Autodesk Inventor part; units mm, degrees
(part 2 of 3)
sketch "Sketch8" plane through (0, 0, 6.35) normal (0, 0, 1) x (1, 0, 0)
  line L0 (-60.6619, -189.7645) -> (-88.5384, -146.9458) projected
  arc A0 (-88.5384, -146.9458) -> (-92.3643, -145.7246) centre (-91.1992, -148.6781) ccw projected
  arc A1 (-96.1321, -146.5792) -> (-92.3643, -145.7246) centre (-97.0248, -133.9106) ccw projected
  arc A2 (-96.1321, -146.5792) -> (-99.0202, -149.1135) centre (-95.909, -149.7463) ccw projected
  line L1 (-99.0202, -149.1135) -> (-103.0485, -168.9169) projected
  arc A3 (-103.0485, -168.9169) -> (-101.38, -172.378) centre (-99.9372, -169.5497) ccw projected
  arc A4 (-94.5438, -182.1572) -> (-101.38, -172.378) centre (-107.1508, -183.6911) ccw projected
  arc A5 (-94.5438, -182.1572) -> (-92.4345, -184.7727) centre (-91.3921, -181.7737) ccw projected
  line L2 (-92.4345, -184.7727) -> (-64.3902, -194.5205) projected
  arc A6 (-64.3902, -194.5205) -> (-61.1133, -193.7771) centre (-63.3478, -191.5215) ccw projected
  arc A7 (-61.0933, -193.7573) -> (-61.1133, -193.7771) centre (-52.1756, -202.7997) ccw projected
  arc A8 (-61.0933, -193.7573) -> (-60.6619, -189.7645) centre (-63.3227, -191.4968) ccw projected
  line L3 (-39.1869, -128.4485) -> (-78.3293, -96.1428) projected
  arc A9 (-86.006, -96.7986) -> (-81.66, -95.6992) centre (-86.8987, -84.1301) ccw projected
  arc A10 (-86.006, -96.7986) -> (-88.8942, -99.3329) centre (-85.7829, -99.9658) ccw projected
  line L4 (-88.8942, -99.3329) -> (-92.9225, -119.1363) projected
  arc A11 (-92.9225, -119.1363) -> (-91.2539, -122.5975) centre (-89.8112, -119.7692) ccw projected
  arc A12 (-85.2508, -129.1499) -> (-91.2539, -122.5975) centre (-97.0248, -133.9106) ccw projected
  arc A13 (-85.2508, -129.1499) -> (-82.5337, -131.1266) centre (-82.3074, -127.9597) ccw projected
  line L5 (-82.5337, -131.1266) -> (-51.925, -133.3143) projected
  arc A14 (-49.8906, -133.4597) -> (-51.925, -133.3143) centre (-51.8103, -146.0138) ccw projected
  line L6 (-49.8906, -133.4597) -> (-41.4343, -134.0641) projected
  arc A15 (-41.4343, -134.0641) -> (-39.1869, -128.4485) centre (-41.2079, -130.8972) ccw projected
  line L7 (-34.396, -142.2066) -> (-35.726, -142.1115) projected
  arc A16 (-35.726, -142.1115) -> (-39.1239, -145.4255) centre (-35.9523, -145.2784) ccw projected
  arc A17 (-46.8246, -157.6942) -> (-39.1239, -145.4255) centre (-51.8103, -146.0138) ccw projected
  line L8 (-46.8246, -157.6942) -> (-63.3432, -164.745) projected
  arc A18 (-63.388, -164.764) -> (-63.3432, -164.745) centre (-68.3289, -153.0646) ccw projected
  arc A19 (-63.388, -164.764) -> (-64.8136, -169.4212) centre (-62.1528, -167.6889) ccw projected
  line L9 (-64.8136, -169.4212) -> (-52.1403, -188.8876) projected
  arc A20 (-52.1403, -188.8876) -> (-50.0187, -190.2842) centre (-49.4795, -187.1553) ccw projected
  arc A21 (-49.6531, -190.3527) -> (-50.0187, -190.2842) centre (-52.1756, -202.7997) ccw projected
  arc A22 (-49.6531, -190.3527) -> (-46.1932, -188.6816) centre (-49.0225, -187.241) ccw projected
  line L10 (-46.1932, -188.6816) -> (-27.8032, -152.5651) projected
  arc A23 (-27.8032, -152.5651) -> (-28.487, -148.784) centre (-30.6326, -151.1244) ccw projected
  arc A24 (-31.6788, -144.1833) -> (-28.487, -148.784) centre (-19.9049, -139.4226) ccw projected
  arc A25 (-31.6788, -144.1833) -> (-34.396, -142.2066) centre (-34.6223, -145.3735) ccw projected
  circle A26 centre (-19.9049, -139.4226) radius 5.588 projected
  circle A27 centre (12.3657, -76.0454) radius 5.588 projected
  circle A28 centre (-52.1756, -202.7997) radius 5.588 projected
  circle A29 centre (-10.4424, -25.9152) radius 6.731 projected
  circle A30 centre (-6.7845, 27.1038) radius 6.731 projected
  line L11 (-56.4256, -250.7609) -> (56.5867, -28.8131) projected
  arc A31 (-133.6537, -223.8049) -> (-56.4256, -250.7609) centre (-93.207, -232.0324) ccw projected
  line L12 (-94.3869, -30.7665) -> (-133.6537, -223.8049) projected
  arc A32 (-79.8174, 0.8875) -> (-94.3869, -30.7665) centre (-19.7161, -45.9556) ccw projected
  line L13 (-50.0844, 39.0359) -> (-79.8174, 0.8875) projected
  arc A33 (56.5867, -28.8131) -> (-50.0844, 39.0359) centre (0, 0) ccw projected
  circle A34 centre (0, 0) radius 13.4937 projected
  line L14 (-92.6277, -239.1082) -> (-87.8938, -227.3235) projected
  arc A35 (-87.8938, -227.3235) -> (-93.7862, -224.9565) centre (-90.84, -226.14) ccw projected
  line L15 (-93.7862, -224.9565) -> (-98.5201, -236.7413) projected
  arc A36 (-98.5201, -236.7413) -> (-92.6277, -239.1082) centre (-95.5739, -237.9247) ccw projected
  circle A37 centre (23.6807, 14.828) radius 6.731 projected
  circle A38 centre (-27.8737, 1.9231) radius 6.731 projected
  circle A39 centre (21.42, -17.9396) radius 6.731 projected
  arc A40 (-106.2582, -196.3597) -> (-98.2131, -192.7137) centre (-107.1508, -183.6911) ccw projected
  arc A41 (-106.2582, -196.3597) -> (-109.1463, -198.894) centre (-106.035, -199.5269) ccw projected
  line L16 (-109.1463, -198.894) -> (-109.9229, -202.7119) projected
  arc A42 (-109.9229, -202.7119) -> (-105.4512, -206.2136) centre (-106.8116, -203.3448) ccw projected
  arc A43 (-67.5559, -219.4407) -> (-76.9832, -208.5096) centre (-93.207, -232.0324) ccw projected
  arc A44 (-67.5559, -219.4407) -> (-61.8764, -219.4822) centre (-64.7057, -218.0416) ccw projected
  line L17 (-61.8764, -219.4822) -> (-60.0739, -215.9422) projected
  arc A45 (-60.0739, -215.9422) -> (-60.7577, -212.1612) centre (-62.9032, -214.5015) ccw projected
  arc A46 (-64.7826, -204.3336) -> (-60.7577, -212.1612) centre (-52.1756, -202.7997) ccw projected
  arc A47 (-64.7826, -204.3336) -> (-66.8919, -201.7181) centre (-67.9343, -204.7171) ccw projected
  line L18 (-66.8919, -201.7181) -> (-72.8348, -199.6524) projected
  arc A48 (-94.9362, -191.9703) -> (-98.2131, -192.7137) centre (-95.9786, -194.9693) ccw projected
  line L19 (-62.2455, -36.9386) -> (-28.8338, -52.5675) projected
  arc A49 (1.0672, -66.5541) -> (4.4031, -66.1517) centre (2.4124, -63.6782) ccw projected
  arc A50 (14.8881, -63.5984) -> (4.4031, -66.1517) centre (12.3657, -76.0454) ccw projected
  arc A51 (14.8881, -63.5984) -> (18.3481, -61.9274) centre (15.5187, -60.4867) ccw projected
  line L20 (18.3481, -61.9274) -> (26.6737, -45.5765) projected
  arc A52 (26.6737, -45.5765) -> (22.3352, -41.3425) centre (23.8443, -44.1359) ccw projected
  arc A53 (-11.2735, -45.6176) -> (22.3352, -41.3425) centre (0, 0) ccw projected
  arc A54 (-46.9122, 2.7029) -> (-52.5862, 4.8373) centre (-50.0819, 2.8855) ccw projected
  line L21 (-52.5862, 4.8373) -> (-64.7921, -10.8233) projected
  arc A55 (-64.7921, -10.8233) -> (-70.5555, -19.8506) centre (-19.7161, -45.9556) ccw projected
  arc A56 (-70.5555, -19.8506) -> (-69.5394, -23.9106) centre (-67.7311, -21.3009) ccw projected
  arc A57 (-64.0747, -34.1201) -> (-69.5394, -23.9106) centre (-76.7726, -34.3495) ccw projected
  arc A58 (-64.0747, -34.1201) -> (-62.2455, -36.9386) centre (-60.9002, -34.0627) ccw projected
  arc A59 (-75.88, -47.0181) -> (-68.81, -44.2433) centre (-76.7726, -34.3495) ccw projected
  arc A60 (-75.88, -47.0181) -> (-78.7681, -49.5524) centre (-75.6568, -50.1853) ccw projected
  line L22 (-78.7681, -49.5524) -> (-82.7964, -69.3558) projected
  arc A61 (-82.7964, -69.3558) -> (-81.1278, -72.8169) centre (-79.6851, -69.9886) ccw projected
  arc A62 (-75.9854, -77.6347) -> (-81.1278, -72.8169) centre (-86.8987, -84.1301) ccw projected
  arc A63 (-75.9854, -77.6347) -> (-72.9993, -79.1754) centre (-73.2571, -76.0109) ccw projected
  line L23 (-72.9993, -79.1754) -> (-14.1778, -74.3847) projected
  arc A64 (-14.1778, -74.3847) -> (-13.0902, -68.3442) centre (-14.4355, -71.2201) ccw projected
  line L24 (-13.0902, -68.3442) -> (-65.4741, -43.8408) projected
  arc A65 (-65.4741, -43.8408) -> (-68.81, -44.2433) centre (-66.8194, -46.7167) ccw projected
  arc A66 (-17.3825, -126.9756) -> (-25.1437, -127.8534) centre (-19.9049, -139.4226) ccw projected
  arc A67 (-17.3825, -126.9756) -> (-13.9226, -125.3045) centre (-16.7519, -123.8638) ccw projected
  line L25 (-13.9226, -125.3045) -> (4.4674, -89.1879) projected
  arc A68 (4.4674, -89.1879) -> (3.7836, -85.4069) centre (1.6381, -87.7473) ccw projected
  arc A69 (1.4524, -82.5408) -> (3.7836, -85.4069) centre (12.3657, -76.0454) ccw projected
  arc A70 (1.4524, -82.5408) -> (-1.5337, -81.0001) centre (-1.2759, -84.1646) ccw projected
  line L26 (-1.5337, -81.0001) -> (-69.4401, -86.5307) projected
  arc A71 (-69.4401, -86.5307) -> (-71.2033, -92.144) centre (-69.1823, -89.6953) ccw projected
  line L27 (-71.2033, -92.144) -> (-28.4744, -127.4098) projected
  arc A72 (-28.4744, -127.4098) -> (-25.1437, -127.8534) centre (-26.4534, -124.9611) ccw projected
  circle A73 centre (-68.3289, -153.0646) radius 6.731 projected
  circle A74 centre (-51.8103, -146.0138) radius 6.731 projected
  line L28 (-76.8234, -201.468) -> (-78.1267, -204.7125) projected
  line L29 (-16.1602, -58.4958) -> (1.0672, -66.5541) projected
  line L30 (-14.9814, -47.5164) -> (-17.7611, -54.4364) projected
  line L31 (-85.1976, -201.8722) -> (-84.1415, -199.2432) projected
  line L32 (-86.0453, -195.0607) -> (-94.9362, -191.9703) projected
  arc A75 (-88.6501, -203.823) -> (-105.4512, -206.2136) centre (-93.207, -232.0324) ccw projected
  line L33 (-24.5423, -50.875) -> (-22.0522, -44.6761) projected
  arc A76 (-46.9122, 2.7029) -> (-23.4162, -40.7399) centre (0, 0) ccw projected
  arc A77 (-72.8348, -199.6524) -> (-76.8234, -201.468) centre (-73.8772, -202.6514) ccw projected
  arc A78 (-78.1267, -204.7125) -> (-76.9832, -208.5096) centre (-75.1805, -205.896) ccw projected
  arc A79 (-11.2735, -45.6176) -> (-14.9814, -47.5164) centre (-12.0352, -48.6999) ccw projected
  arc A80 (-17.7611, -54.4364) -> (-16.1602, -58.4958) centre (-14.8149, -55.6198) ccw projected
  arc A81 (-78.3293, -96.1428) -> (-81.66, -95.6992) centre (-80.3503, -98.5915) ccw projected
  arc A82 (-84.1415, -199.2432) -> (-86.0453, -195.0607) centre (-87.0877, -198.0597) ccw projected
  arc A83 (-88.6501, -203.823) -> (-85.1976, -201.8722) centre (-88.1438, -200.6887) ccw projected
  arc A84 (-22.0522, -44.6761) -> (-23.4162, -40.7399) centre (-24.9984, -43.4926) ccw projected
  arc A85 (-28.8338, -52.5675) -> (-24.5423, -50.875) centre (-27.4885, -49.6916) ccw projected
  point P0 (0, 0)
  point P1 (-93.2076, -232.0321)
  point P2 (0, 0)
extrude "Extrusion8" cut sketch "Sketch8" against normal blind 6.35 contours A8 A7 A6 L2 A5 A4 A3 L1 A2 A1 A0 L0 | A40 A48 L32 A82 L31 A83 A75 A42 L16 A41 | A43 A78 L28 A77 L18 A47 A46 A45 L17 A44 | A58 A57 A56 A55 L21 A54 A76 A84 L33 A85 L19 | L29 A80 L30 A79 A53 A52 L20 A51 A50 A49 | A59 A65 L24 A64 L23 A63 A62 A61 L22 A60 | A66 A72 L27 A71 L26 A70 A69 A68 L25 A67
sketch "Sketch9" plane through (0, 0, 6.35) normal (0, 0, 1) x (1, 0, 0)
  arc A0 (-88.6501, -203.823) -> (-105.4512, -206.2136) centre (-93.207, -232.0324) ccw projected
  arc A1 (-109.9229, -202.7119) -> (-105.4512, -206.2136) centre (-106.8116, -203.3448) ccw projected
  line L0 (-109.9229, -202.7119) -> (-109.1463, -198.894) projected
  arc A2 (-106.2582, -196.3597) -> (-109.1463, -198.894) centre (-106.035, -199.5269) ccw projected
  arc A3 (-106.2582, -196.3597) -> (-98.2131, -192.7137) centre (-107.1508, -183.6911) ccw projected
  arc A4 (-94.9362, -191.9703) -> (-98.2131, -192.7137) centre (-95.9786, -194.9693) ccw projected
  line L1 (-94.9362, -191.9703) -> (-86.0453, -195.0607) projected
  arc A5 (-84.1415, -199.2432) -> (-86.0453, -195.0607) centre (-87.0877, -198.0597) ccw projected
  line L2 (-84.1415, -199.2432) -> (-85.1976, -201.8722) projected
  arc A6 (-88.6501, -203.823) -> (-85.1976, -201.8722) centre (-88.1438, -200.6887) ccw projected
  arc A7 (-28.8338, -52.5675) -> (-24.5423, -50.875) centre (-27.4885, -49.6916) ccw projected
  line L3 (-28.8338, -52.5675) -> (-62.2455, -36.9386) projected
  arc A8 (-64.0747, -34.1201) -> (-62.2455, -36.9386) centre (-60.9002, -34.0627) ccw projected
  arc A9 (-64.0747, -34.1201) -> (-69.5394, -23.9106) centre (-76.7726, -34.3495) ccw projected
  arc A10 (-70.5555, -19.8506) -> (-69.5394, -23.9106) centre (-67.7311, -21.3009) ccw projected
  arc A11 (-64.7921, -10.8233) -> (-70.5555, -19.8506) centre (-19.7161, -45.9556) ccw projected
  line L4 (-64.7921, -10.8233) -> (-52.5862, 4.8373) projected
  arc A12 (-46.9122, 2.7029) -> (-52.5862, 4.8373) centre (-50.0819, 2.8855) ccw projected
  arc A13 (-46.9122, 2.7029) -> (-23.4162, -40.7399) centre (0, 0) ccw projected
  arc A14 (-22.0522, -44.6761) -> (-23.4162, -40.7399) centre (-24.9984, -43.4926) ccw projected
  line L5 (-22.0522, -44.6761) -> (-24.5423, -50.875) projected
  arc A15 (-88.5384, -146.9458) -> (-92.3643, -145.7246) centre (-91.1992, -148.6781) ccw projected
  line L6 (-88.5384, -146.9458) -> (-60.6619, -189.7645) projected
  arc A16 (-61.0933, -193.7573) -> (-60.6619, -189.7645) centre (-63.3227, -191.4968) ccw projected
  arc A17 (-61.0933, -193.7573) -> (-61.1133, -193.7771) centre (-52.1756, -202.7997) ccw projected
  arc A18 (-64.3902, -194.5205) -> (-61.1133, -193.7771) centre (-63.3478, -191.5215) ccw projected
  line L7 (-64.3902, -194.5205) -> (-92.4345, -184.7727) projected
  arc A19 (-94.5438, -182.1572) -> (-92.4345, -184.7727) centre (-91.3921, -181.7737) ccw projected
  arc A20 (-94.5438, -182.1572) -> (-101.38, -172.378) centre (-107.1508, -183.6911) ccw projected
  arc A21 (-103.0485, -168.9169) -> (-101.38, -172.378) centre (-99.9372, -169.5497) ccw projected
  line L8 (-103.0485, -168.9169) -> (-99.0202, -149.1135) projected
  arc A22 (-96.1321, -146.5792) -> (-99.0202, -149.1135) centre (-95.909, -149.7463) ccw projected
  arc A23 (-96.1321, -146.5792) -> (-92.3643, -145.7246) centre (-97.0248, -133.9106) ccw projected
  arc A24 (-17.7611, -54.4364) -> (-16.1602, -58.4958) centre (-14.8149, -55.6198) ccw projected
  line L9 (-17.7611, -54.4364) -> (-14.9814, -47.5164) projected
  arc A25 (-11.2735, -45.6176) -> (-14.9814, -47.5164) centre (-12.0352, -48.6999) ccw projected
  arc A26 (-11.2735, -45.6176) -> (22.3352, -41.3425) centre (0, 0) ccw projected
  arc A27 (26.6737, -45.5765) -> (22.3352, -41.3425) centre (23.8443, -44.1359) ccw projected
  line L10 (26.6737, -45.5765) -> (18.3481, -61.9274) projected
  arc A28 (14.8881, -63.5984) -> (18.3481, -61.9274) centre (15.5187, -60.4867) ccw projected
  arc A29 (14.8881, -63.5984) -> (4.4031, -66.1517) centre (12.3657, -76.0454) ccw projected
  arc A30 (1.0672, -66.5541) -> (4.4031, -66.1517) centre (2.4124, -63.6782) ccw projected
  line L11 (1.0672, -66.5541) -> (-16.1602, -58.4958) projected
  arc A31 (-75.9854, -77.6347) -> (-81.1278, -72.8169) centre (-86.8987, -84.1301) ccw projected
  arc A32 (-82.7964, -69.3558) -> (-81.1278, -72.8169) centre (-79.6851, -69.9886) ccw projected
  line L12 (-82.7964, -69.3558) -> (-78.7681, -49.5524) projected
  arc A33 (-75.88, -47.0181) -> (-78.7681, -49.5524) centre (-75.6568, -50.1853) ccw projected
  arc A34 (-75.88, -47.0181) -> (-68.81, -44.2433) centre (-76.7726, -34.3495) ccw projected
  arc A35 (-65.4741, -43.8408) -> (-68.81, -44.2433) centre (-66.8194, -46.7167) ccw projected
  line L13 (-65.4741, -43.8408) -> (-13.0902, -68.3442) projected
  arc A36 (-14.1778, -74.3847) -> (-13.0902, -68.3442) centre (-14.4355, -71.2201) ccw projected
  line L14 (-14.1778, -74.3847) -> (-72.9993, -79.1754) projected
  arc A37 (-75.9854, -77.6347) -> (-72.9993, -79.1754) centre (-73.2571, -76.0109) ccw projected
  arc A38 (1.4524, -82.5408) -> (3.7836, -85.4069) centre (12.3657, -76.0454) ccw projected
  arc A39 (4.4674, -89.1879) -> (3.7836, -85.4069) centre (1.6381, -87.7473) ccw projected
  line L15 (4.4674, -89.1879) -> (-13.9226, -125.3045) projected
  arc A40 (-17.3825, -126.9756) -> (-13.9226, -125.3045) centre (-16.7519, -123.8638) ccw projected
  arc A41 (-17.3825, -126.9756) -> (-25.1437, -127.8534) centre (-19.9049, -139.4226) ccw projected
  arc A42 (-28.4744, -127.4098) -> (-25.1437, -127.8534) centre (-26.4534, -124.9611) ccw projected
  line L16 (-28.4744, -127.4098) -> (-71.2033, -92.144) projected
  arc A43 (-69.4401, -86.5307) -> (-71.2033, -92.144) centre (-69.1823, -89.6953) ccw projected
  line L17 (-69.4401, -86.5307) -> (-1.5337, -81.0001) projected
  arc A44 (1.4524, -82.5408) -> (-1.5337, -81.0001) centre (-1.2759, -84.1646) ccw projected
  arc A45 (-64.7826, -204.3336) -> (-60.7577, -212.1612) centre (-52.1756, -202.7997) ccw projected
  arc A46 (-60.0739, -215.9422) -> (-60.7577, -212.1612) centre (-62.9032, -214.5015) ccw projected
  line L18 (-60.0739, -215.9422) -> (-61.8764, -219.4822) projected
  arc A47 (-67.5559, -219.4407) -> (-61.8764, -219.4822) centre (-64.7057, -218.0416) ccw projected
  arc A48 (-67.5559, -219.4407) -> (-76.9832, -208.5096) centre (-93.207, -232.0324) ccw projected
  arc A49 (-78.1267, -204.7125) -> (-76.9832, -208.5096) centre (-75.1805, -205.896) ccw projected
  line L19 (-78.1267, -204.7125) -> (-76.8234, -201.468) projected
  arc A50 (-72.8348, -199.6524) -> (-76.8234, -201.468) centre (-73.8772, -202.6514) ccw projected
  line L20 (-72.8348, -199.6524) -> (-66.8919, -201.7181) projected
  arc A51 (-64.7826, -204.3336) -> (-66.8919, -201.7181) centre (-67.9343, -204.7171) ccw projected
  circle A52 centre (-19.9049, -139.4226) radius 5.588 projected
  circle A53 centre (-107.1541, -183.6919) radius 5.588 projected
  circle A54 centre (-86.902, -84.1308) radius 5.588 projected
  circle A55 centre (-56.5442, -157.7985) radius 6.731 projected
  line L21 (-98.5201, -236.7413) -> (-93.7862, -224.9565) projected
  arc A56 (-87.8938, -227.3235) -> (-93.7862, -224.9565) centre (-90.84, -226.14) ccw projected
  line L22 (-87.8938, -227.3235) -> (-92.6277, -239.1082) projected
  arc A57 (-98.5201, -236.7413) -> (-92.6277, -239.1082) centre (-95.5739, -237.9247) ccw projected
  circle A58 centre (0, 0) radius 13.4937 projected
  arc A59 (56.5867, -28.8131) -> (-50.0844, 39.0359) centre (0, 0) ccw projected
  line L23 (-50.0844, 39.0359) -> (-79.8174, 0.8875) projected
  arc A60 (-79.8174, 0.8875) -> (-94.3869, -30.7665) centre (-19.7161, -45.9556) ccw projected
  line L24 (-94.3869, -30.7665) -> (-133.6537, -223.8049) projected
  arc A61 (-133.6537, -223.8049) -> (-56.4256, -250.7609) centre (-93.207, -232.0324) ccw projected
  line L25 (-56.4256, -250.7609) -> (56.5867, -28.8131) projected
  circle A62 centre (-63.595, -141.2799) radius 6.731 projected
  arc A63 (-11.6087, -28.8683) -> (-9.2396, -22.9769) centre (-10.4059, -25.9299) ccw projected
  arc A64 (-9.2396, -22.9769) -> (-11.6087, -28.8683) centre (-10.4424, -25.9152) ccw projected
  arc A65 (26.36, 16.5315) -> (20.9805, 13.1578) centre (23.6598, 14.8613) ccw projected
  arc A66 (20.9805, 13.1578) -> (26.36, 16.5315) centre (23.6807, 14.828) ccw projected
  arc A67 (23.8681, -19.9613) -> (18.9971, -15.8876) centre (21.4452, -17.9094) ccw projected
  arc A68 (18.9971, -15.8876) -> (23.8681, -19.9613) centre (21.42, -17.9396) ccw projected
  arc A69 (-7.5767, 30.1783) -> (-6.0305, 24.0196) centre (-6.8227, 27.0942) ccw projected
  arc A70 (-6.0305, 24.0196) -> (-7.5767, 30.1783) centre (-6.7845, 27.1038) ccw projected
  arc A71 (-31.0426, 2.1197) -> (-24.7075, 1.6871) centre (-27.8764, 1.8838) ccw projected
  arc A72 (-24.7075, 1.6871) -> (-31.0426, 2.1197) centre (-27.8737, 1.9231) ccw projected
  circle A73 centre (-76.7759, -34.3502) radius 5.588 projected
  circle A74 centre (-97.0281, -133.9113) radius 5.588 projected
  circle A75 centre (12.3657, -76.0454) radius 5.588 projected
  circle A76 centre (-52.1756, -202.7997) radius 5.588 projected
  circle A77 centre (-56.5442, -157.7985) radius 3.175 projected
  circle A78 centre (-56.5442, -157.7985) radius 12.7
  circle A79 centre (-63.595, -141.2799) radius 12.7
  line L26 (-68.2246, -162.7842) -> (-75.2755, -146.2655)
  line L27 (-51.9146, -136.2942) -> (-44.8637, -152.8128)
  circle A80 centre (-19.9049, -139.4226) radius 2.413 projected
  circle A81 centre (-97.0281, -133.9113) radius 2.413 projected
  line L28 (-19.9049, -139.4226) -> (-97.0281, -133.9113)
  circle A82 centre (-52.1756, -202.7997) radius 2.413 projected
  line L29 (-97.0281, -133.9113) -> (-52.1756, -202.7997)
  line L30 (-57.469, -187.6858) -> (-85.3454, -144.8671)
  arc A83 (-85.3454, -144.8671) -> (-93.7625, -142.1804) centre (-91.1992, -148.6781) ccw
  arc A84 (-96.3999, -142.7786) -> (-93.7625, -142.1804) centre (-97.0248, -133.9106) ccw
  arc A85 (-96.3999, -142.7786) -> (-102.7538, -148.354) centre (-95.909, -149.7463) ccw
  line L31 (-102.7538, -148.354) -> (-106.7821, -168.1574)
  arc A86 (-106.7821, -168.1574) -> (-103.1112, -175.772) centre (-99.9372, -169.5497) ccw
  arc A87 (-98.3259, -182.6174) -> (-103.1112, -175.772) centre (-107.1508, -183.6911) ccw
  arc A88 (-98.3259, -182.6174) -> (-93.6854, -188.3715) centre (-91.3921, -181.7737) ccw
  line L32 (-93.6854, -188.3715) -> (-65.641, -198.1193)
  arc A89 (-65.641, -198.1193) -> (-58.432, -196.4839) centre (-63.3478, -191.5215) ccw
  arc A90 (-58.418, -196.47) -> (-58.432, -196.4839) centre (-52.1756, -202.7997) ccw
  arc A91 (-58.418, -196.47) -> (-57.469, -187.6858) centre (-63.3227, -191.4968) ccw
  line L33 (-19.647, -135.6213) -> (-104.4046, -129.5645)
  line L34 (-104.4046, -129.5645) -> (-55.3622, -204.8881)
  line L35 (-20.1902, -143.2219) -> (-89.6515, -138.2582)
  line L36 (-89.6515, -138.2582) -> (-48.9765, -200.7304)
  arc A92 (39.6107, -20.1691) -> (-35.0591, 27.3251) centre (0, 0) ccw
  line L37 (-35.0591, 27.3251) -> (-64.7921, -10.8233)
  arc A93 (-64.7921, -10.8233) -> (-75.7192, -34.5638) centre (-19.7161, -45.9556) ccw
  line L38 (-75.7192, -34.5638) -> (-114.986, -227.6022)
  arc A94 (-114.986, -227.6022) -> (-73.4016, -242.1169) centre (-93.207, -232.0324) ccw
  line L39 (-73.4016, -242.1169) -> (39.6107, -20.1691)
  line L40 (-76.0538, -98.0209) -> (-33.3248, -133.2867)
  arc A95 (-33.3248, -133.2867) -> (-22.0004, -134.7949) centre (-26.4534, -124.9611) ccw
  arc A96 (-18.896, -134.4438) -> (-22.0004, -134.7949) centre (-19.9049, -139.4226) ccw
  arc A97 (-18.896, -134.4438) -> (-7.1321, -128.762) centre (-16.7519, -123.8638) ccw
  line L41 (-7.1321, -128.762) -> (11.2578, -92.6455)
  arc A98 (11.2578, -92.6455) -> (8.9329, -79.79) centre (1.6381, -87.7473) ccw
  arc A99 (8.0004, -78.6436) -> (8.9329, -79.79) centre (12.3657, -76.0454) ccw
  arc A100 (8.0004, -78.6436) -> (-2.1522, -73.4052) centre (-1.2759, -84.1646) ccw
  line L42 (-2.1522, -73.4052) -> (-70.0586, -78.9359)
  arc A101 (-70.0586, -78.9359) -> (-76.0538, -98.0209) centre (-69.1823, -89.6953) ccw
  spline S0 degree 4 poles (-63.6057, -178.2615) (-65.5406, -175.2881) (-67.0528, -169.1426) (-60.675, -170.3492) (-57.0315, -170.4891) knots 0 0 0 0 0 1 1 1 1 1
  circle A102 centre (-52.1756, -202.7997) radius 12.7002
  circle A103 centre (-56.5442, -157.7985) radius 3.175 projected
  spline S1 degree 1 poles (-56.5442, -157.7985) (-35.8368, -168.3424) knots 0 0 1 1
  circle A104 centre (-19.9049, -139.4226) radius 12.6998
  spline S2 degree 3 poles (-54.8154, -154.4033) (-47.9129, -157.9179) (-41.0105, -161.4326) (-34.108, -164.9472) knots 0 0 0 0 1 1 1 1
  spline S3 degree 3 poles (-58.273, -161.1937) (-51.3705, -164.7083) (-44.468, -168.223) (-37.5656, -171.7376) knots 0 0 0 0 1 1 1 1
  point P0 (0, 0)
  point P1 (-64.3688, -171.7862)
  point P2 (-47.4769, -166.6909)
  point P3 (-55.5931, -190.5679)
  point P4 (-47.3915, -191.035)
  point P5 (-26.6047, -150.2113)
  point P6 (-32.2605, -142.3593)
  point P7 (-49.8626, -141.1015)
  point P8 (-44.0194, -159.9005)
  point P9 (-34.108, -164.9472)
  dimension "d37" = 3.81
  dimension "d38" = 3.81
  dimension "d30" = 25.4
  dimension "d31" = 25.4
  dimension "d32" = 3.81
  dimension "d33" = 3.81
  dimension "d34" = 3.81
  dimension "d35" = 19.05
  dimension "d36" = 7.62
  constraints: 43 point on circle, 34 end point, 23 centre point, 4 coincident, 3 point on line, 3 tangent, 1 parallel, 40 other
  measures "d30" diameter of A78
  measures "d31" diameter of A79
  measures "d32" distance between parallel lines of L6 L30
  measures "d33" distance between parallel lines of L28 L33
  measures "d34" distance between parallel lines of L28 L35
  measures "d35" distance between parallel lines of L25 L39
  measures "d36" distance between parallel lines of L16 L40
extrude "Extrusion9" cut sketch "Sketch9" against normal blind 6.35 contours A102 L36 L30 S0 A78 S3 L39 | S2 A78 L27 L35 A104 L39
fillet "Fillet1" radius 3.175 9 edges at (-49.8626, -141.1015, 3.175) (-32.2605, -142.3593, 3.175) (-26.6047, -150.2113, 3.175) (-44.0194, -159.9005, 3.175) (-34.108, -164.9472, 3.175) (-37.5656, -171.7376, 3.175) (-47.4769, -166.6909, 3.175) (-47.3915, -191.035, 3.175) (-55.5931, -190.5679, 3.175)
sketch "Sketch10" plane through (0, 0, 6.35) normal (0, 0, 1) x (1, 0, 0)
  arc A0 (-57.0315, -170.4891) -> (-48.9168, -167.9529) centre (-56.5442, -157.7985) ccw projected
  arc A1 (-45.5693, -167.6622) -> (-48.9168, -167.9529) centre (-47.0099, -170.4916) ccw projected
  line L0 (-45.5693, -167.6622) -> (-40.3949, -170.2969) projected
  arc A2 (-39.0062, -174.5669) -> (-40.3949, -170.2969) centre (-41.8356, -173.1263) ccw projected
  line L1 (-39.0062, -174.5669) -> (-46.1931, -188.6814) projected
  arc A3 (-49.6531, -190.3525) -> (-46.1931, -188.6814) centre (-49.0224, -187.2408) ccw projected
  arc A4 (-49.6531, -190.3525) -> (-53.7154, -190.1932) centre (-52.1756, -202.7997) ccw projected
  arc A5 (-56.7611, -188.774) -> (-53.7154, -190.1932) centre (-54.1004, -187.0416) ccw projected
  line L2 (-56.7611, -188.774) -> (-63.6057, -178.2615) projected
  line L3 (-44.8637, -152.8128) -> (-47.8206, -145.8856) projected
  arc A6 (-44.6741, -141.4723) -> (-47.8206, -145.8856) centre (-44.9004, -144.6392) ccw projected
  line L4 (-44.6741, -141.4723) -> (-34.3957, -142.2068) projected
  arc A7 (-31.6785, -144.1834) -> (-34.3957, -142.2068) centre (-34.622, -145.3737) ccw projected
  arc A8 (-31.6785, -144.1834) -> (-28.4869, -148.7838) centre (-19.9049, -139.4226) ccw projected
  arc A9 (-27.8031, -152.5648) -> (-28.4869, -148.7838) centre (-30.6324, -151.1242) ccw projected
  line L5 (-27.8031, -152.5648) -> (-32.6673, -162.1179) projected
  arc A10 (-36.9373, -163.5065) -> (-32.6673, -162.1179) centre (-35.4967, -160.6772) ccw projected
  line L6 (-36.9373, -163.5065) -> (-42.1117, -160.8718) projected
  arc A11 (-43.8457, -157.9937) -> (-42.1117, -160.8718) centre (-40.6711, -158.0425) ccw projected
  arc A12 (-43.8457, -157.9937) -> (-44.8637, -152.8128) centre (-56.5442, -157.7985) ccw projected
  arc A13 (-88.6501, -203.823) -> (-105.4512, -206.2136) centre (-93.207, -232.0324) ccw projected
  arc A14 (-109.9229, -202.7119) -> (-105.4512, -206.2136) centre (-106.8116, -203.3448) ccw projected
  line L7 (-109.9229, -202.7119) -> (-109.1463, -198.894) projected
  arc A15 (-106.2582, -196.3597) -> (-109.1463, -198.894) centre (-106.035, -199.5269) ccw projected
  arc A16 (-106.2582, -196.3597) -> (-98.2131, -192.7137) centre (-107.1508, -183.6911) ccw projected
  arc A17 (-94.9362, -191.9703) -> (-98.2131, -192.7137) centre (-95.9786, -194.9693) ccw projected
  line L8 (-94.9362, -191.9703) -> (-86.0453, -195.0607) projected
  arc A18 (-84.1415, -199.2432) -> (-86.0453, -195.0607) centre (-87.0877, -198.0597) ccw projected
  line L9 (-84.1415, -199.2432) -> (-85.1976, -201.8722) projected
  arc A19 (-88.6501, -203.823) -> (-85.1976, -201.8722) centre (-88.1438, -200.6887) ccw projected
  arc A20 (-28.8338, -52.5675) -> (-24.5423, -50.875) centre (-27.4885, -49.6916) ccw projected
  line L10 (-28.8338, -52.5675) -> (-62.2455, -36.9386) projected
  arc A21 (-64.0747, -34.1201) -> (-62.2455, -36.9386) centre (-60.9002, -34.0627) ccw projected
  arc A22 (-64.0747, -34.1201) -> (-69.5394, -23.9106) centre (-76.7726, -34.3495) ccw projected
  arc A23 (-70.5555, -19.8506) -> (-69.5394, -23.9106) centre (-67.7311, -21.3009) ccw projected
  arc A24 (-64.7921, -10.8233) -> (-70.5555, -19.8506) centre (-19.7161, -45.9556) ccw projected
  line L11 (-64.7921, -10.8233) -> (-52.5862, 4.8373) projected
  arc A25 (-46.9122, 2.7029) -> (-52.5862, 4.8373) centre (-50.0819, 2.8855) ccw projected
  arc A26 (-46.9122, 2.7029) -> (-23.4162, -40.7399) centre (0, 0) ccw projected
  arc A27 (-22.0522, -44.6761) -> (-23.4162, -40.7399) centre (-24.9984, -43.4926) ccw projected
  line L12 (-22.0522, -44.6761) -> (-24.5423, -50.875) projected
  arc A28 (-88.5384, -146.9458) -> (-92.3643, -145.7246) centre (-91.1992, -148.6781) ccw projected
  line L13 (-88.5384, -146.9458) -> (-60.6619, -189.7645) projected
  arc A29 (-61.0933, -193.7573) -> (-60.6619, -189.7645) centre (-63.3227, -191.4968) ccw projected
  arc A30 (-61.0933, -193.7573) -> (-61.1133, -193.7771) centre (-52.1756, -202.7997) ccw projected
  arc A31 (-64.3902, -194.5205) -> (-61.1133, -193.7771) centre (-63.3478, -191.5215) ccw projected
  line L14 (-64.3902, -194.5205) -> (-92.4345, -184.7727) projected
  arc A32 (-94.5438, -182.1572) -> (-92.4345, -184.7727) centre (-91.3921, -181.7737) ccw projected
  arc A33 (-94.5438, -182.1572) -> (-101.38, -172.378) centre (-107.1508, -183.6911) ccw projected
  arc A34 (-103.0485, -168.9169) -> (-101.38, -172.378) centre (-99.9372, -169.5497) ccw projected
  line L15 (-103.0485, -168.9169) -> (-99.0202, -149.1135) projected
  arc A35 (-96.1321, -146.5792) -> (-99.0202, -149.1135) centre (-95.909, -149.7463) ccw projected
  arc A36 (-96.1321, -146.5792) -> (-92.3643, -145.7246) centre (-97.0248, -133.9106) ccw projected
  arc A37 (-17.7611, -54.4364) -> (-16.1602, -58.4958) centre (-14.8149, -55.6198) ccw projected
  line L16 (-17.7611, -54.4364) -> (-14.9814, -47.5164) projected
  arc A38 (-11.2735, -45.6176) -> (-14.9814, -47.5164) centre (-12.0352, -48.6999) ccw projected
  arc A39 (-11.2735, -45.6176) -> (22.3352, -41.3425) centre (0, 0) ccw projected
  arc A40 (26.6737, -45.5765) -> (22.3352, -41.3425) centre (23.8443, -44.1359) ccw projected
  line L17 (26.6737, -45.5765) -> (18.3481, -61.9274) projected
  arc A41 (14.8881, -63.5984) -> (18.3481, -61.9274) centre (15.5187, -60.4867) ccw projected
  arc A42 (14.8881, -63.5984) -> (4.4031, -66.1517) centre (12.3657, -76.0454) ccw projected
  arc A43 (1.0672, -66.5541) -> (4.4031, -66.1517) centre (2.4124, -63.6782) ccw projected
  line L18 (1.0672, -66.5541) -> (-16.1602, -58.4958) projected
  arc A44 (-75.9854, -77.6347) -> (-81.1278, -72.8169) centre (-86.8987, -84.1301) ccw projected
  arc A45 (-82.7964, -69.3558) -> (-81.1278, -72.8169) centre (-79.6851, -69.9886) ccw projected
  line L19 (-82.7964, -69.3558) -> (-78.7681, -49.5524) projected
  arc A46 (-75.88, -47.0181) -> (-78.7681, -49.5524) centre (-75.6568, -50.1853) ccw projected
  arc A47 (-75.88, -47.0181) -> (-68.81, -44.2433) centre (-76.7726, -34.3495) ccw projected
  arc A48 (-65.4741, -43.8408) -> (-68.81, -44.2433) centre (-66.8194, -46.7167) ccw projected
  line L20 (-65.4741, -43.8408) -> (-13.0902, -68.3442) projected
  arc A49 (-14.1778, -74.3847) -> (-13.0902, -68.3442) centre (-14.4355, -71.2201) ccw projected
  line L21 (-14.1778, -74.3847) -> (-72.9993, -79.1754) projected
  arc A50 (-75.9854, -77.6347) -> (-72.9993, -79.1754) centre (-73.2571, -76.0109) ccw projected
  arc A51 (1.4524, -82.5408) -> (3.7836, -85.4069) centre (12.3657, -76.0454) ccw projected
  arc A52 (4.4674, -89.1879) -> (3.7836, -85.4069) centre (1.6381, -87.7473) ccw projected
  line L22 (4.4674, -89.1879) -> (-13.9226, -125.3045) projected
  arc A53 (-17.3825, -126.9756) -> (-13.9226, -125.3045) centre (-16.7519, -123.8638) ccw projected
  arc A54 (-17.3825, -126.9756) -> (-25.1437, -127.8534) centre (-19.9049, -139.4226) ccw projected
  arc A55 (-28.4744, -127.4098) -> (-25.1437, -127.8534) centre (-26.4534, -124.9611) ccw projected
  line L23 (-28.4744, -127.4098) -> (-71.2033, -92.144) projected
  arc A56 (-69.4401, -86.5307) -> (-71.2033, -92.144) centre (-69.1823, -89.6953) ccw projected
  line L24 (-69.4401, -86.5307) -> (-1.5337, -81.0001) projected
  arc A57 (1.4524, -82.5408) -> (-1.5337, -81.0001) centre (-1.2759, -84.1646) ccw projected
  arc A58 (-64.7826, -204.3336) -> (-60.7577, -212.1612) centre (-52.1756, -202.7997) ccw projected
  arc A59 (-60.0739, -215.9422) -> (-60.7577, -212.1612) centre (-62.9032, -214.5015) ccw projected
  line L25 (-60.0739, -215.9422) -> (-61.8764, -219.4822) projected
  arc A60 (-67.5559, -219.4407) -> (-61.8764, -219.4822) centre (-64.7057, -218.0416) ccw projected
  arc A61 (-67.5559, -219.4407) -> (-76.9832, -208.5096) centre (-93.207, -232.0324) ccw projected
  arc A62 (-78.1267, -204.7125) -> (-76.9832, -208.5096) centre (-75.1805, -205.896) ccw projected
  line L26 (-78.1267, -204.7125) -> (-76.8234, -201.468) projected
  arc A63 (-72.8348, -199.6524) -> (-76.8234, -201.468) centre (-73.8772, -202.6514) ccw projected
  line L27 (-72.8348, -199.6524) -> (-66.8919, -201.7181) projected
  arc A64 (-64.7826, -204.3336) -> (-66.8919, -201.7181) centre (-67.9343, -204.7171) ccw projected
  circle A65 centre (-19.9049, -139.4226) radius 5.588 projected
  circle A66 centre (-107.1541, -183.6919) radius 5.588 projected
  circle A67 centre (-86.902, -84.1308) radius 5.588 projected
  circle A68 centre (-56.5442, -157.7985) radius 6.731 projected
  line L28 (-98.5201, -236.7413) -> (-93.7862, -224.9565) projected
  arc A69 (-87.8938, -227.3235) -> (-93.7862, -224.9565) centre (-90.84, -226.14) ccw projected
  line L29 (-87.8938, -227.3235) -> (-92.6277, -239.1082) projected
  arc A70 (-98.5201, -236.7413) -> (-92.6277, -239.1082) centre (-95.5739, -237.9247) ccw projected
  circle A71 centre (0, 0) radius 13.4937 projected
  arc A72 (56.5867, -28.8131) -> (-50.0844, 39.0359) centre (0, 0) ccw projected
  line L30 (-50.0844, 39.0359) -> (-79.8174, 0.8875) projected
  arc A73 (-79.8174, 0.8875) -> (-94.3869, -30.7665) centre (-19.7161, -45.9556) ccw projected
  line L31 (-94.3869, -30.7665) -> (-133.6537, -223.8049) projected
  arc A74 (-133.6537, -223.8049) -> (-56.4256, -250.7609) centre (-93.207, -232.0324) ccw projected
  line L32 (-56.4256, -250.7609) -> (56.5867, -28.8131) projected
  circle A75 centre (-63.595, -141.2799) radius 6.731 projected
  arc A76 (-11.6087, -28.8683) -> (-9.2396, -22.9769) centre (-10.4059, -25.9299) ccw projected
  arc A77 (-9.2396, -22.9769) -> (-11.6087, -28.8683) centre (-10.4424, -25.9152) ccw projected
  arc A78 (26.36, 16.5315) -> (20.9805, 13.1578) centre (23.6598, 14.8613) ccw projected
  arc A79 (20.9805, 13.1578) -> (26.36, 16.5315) centre (23.6807, 14.828) ccw projected
  arc A80 (23.8681, -19.9613) -> (18.9971, -15.8876) centre (21.4452, -17.9094) ccw projected
  arc A81 (18.9971, -15.8876) -> (23.8681, -19.9613) centre (21.42, -17.9396) ccw projected
  arc A82 (-7.5767, 30.1783) -> (-6.0305, 24.0196) centre (-6.8227, 27.0942) ccw projected
  arc A83 (-6.0305, 24.0196) -> (-7.5767, 30.1783) centre (-6.7845, 27.1038) ccw projected
  arc A84 (-31.0426, 2.1197) -> (-24.7075, 1.6871) centre (-27.8764, 1.8838) ccw projected
  arc A85 (-24.7075, 1.6871) -> (-31.0426, 2.1197) centre (-27.8737, 1.9231) ccw projected
  circle A86 centre (-76.7759, -34.3502) radius 5.588 projected
  circle A87 centre (-97.0281, -133.9113) radius 5.588 projected
  circle A88 centre (12.3657, -76.0454) radius 5.588 projected
  circle A89 centre (-52.1756, -202.7997) radius 5.588 projected
  line L33 (-76.0538, -98.0209) -> (-33.3248, -133.2867)
  arc A90 (-33.3248, -133.2867) -> (-22.0004, -134.7949) centre (-26.4534, -124.9611) ccw
  arc A91 (-18.896, -134.4438) -> (-22.0004, -134.7949) centre (-19.9049, -139.4226) ccw
  arc A92 (-18.896, -134.4438) -> (-7.1321, -128.762) centre (-16.7519, -123.8638) ccw
  line L34 (-7.1321, -128.762) -> (11.2578, -92.6455)
  arc A93 (11.2578, -92.6455) -> (8.9329, -79.79) centre (1.6381, -87.7473) ccw
  arc A94 (8.0004, -78.6436) -> (8.9329, -79.79) centre (12.3657, -76.0454) ccw
  arc A95 (8.0004, -78.6436) -> (-2.1522, -73.4052) centre (-1.2759, -84.1646) ccw
  line L35 (-2.1522, -73.4052) -> (-70.0586, -78.9359)
  arc A96 (-70.0586, -78.9359) -> (-76.0538, -98.0209) centre (-69.1823, -89.6953) ccw
  line L36 (-54.276, -185.607) -> (-82.1525, -142.7883)
  arc A97 (-82.1525, -142.7883) -> (-95.1606, -138.6362) centre (-91.1992, -148.6781) ccw
  arc A98 (-96.6677, -138.978) -> (-95.1606, -138.6362) centre (-97.0248, -133.9106) ccw
  arc A99 (-96.6677, -138.978) -> (-106.4873, -147.5946) centre (-95.909, -149.7463) ccw
  line L37 (-106.4873, -147.5946) -> (-110.5156, -167.3979)
  arc A100 (-110.5156, -167.3979) -> (-104.8425, -179.1659) centre (-99.9372, -169.5497) ccw
  arc A101 (-102.108, -183.0776) -> (-104.8425, -179.1659) centre (-107.1508, -183.6911) ccw
  arc A102 (-102.108, -183.0776) -> (-94.9362, -191.9703) centre (-91.3921, -181.7737) ccw
  line L38 (-94.9362, -191.9703) -> (-66.8919, -201.7181)
  arc A103 (-66.8919, -201.7181) -> (-55.7507, -199.1907) centre (-63.3478, -191.5215) ccw
  arc A104 (-55.7427, -199.1827) -> (-55.7507, -199.1907) centre (-52.1756, -202.7997) ccw
  arc A105 (-55.7427, -199.1827) -> (-54.276, -185.607) centre (-63.3227, -191.4968) ccw
  line L39 (-114.986, -227.6022) -> (-75.7192, -34.5638)
  arc A106 (-64.7921, -10.8233) -> (-75.7192, -34.5638) centre (-19.7161, -45.9556) ccw
  line L40 (-64.7921, -10.8233) -> (-35.0591, 27.3251)
  arc A107 (39.6107, -20.1691) -> (-35.0591, 27.3251) centre (0, 0) ccw
  line L41 (39.6107, -20.1691) -> (-73.4016, -242.1169)
  arc A108 (-114.986, -227.6022) -> (-73.4016, -242.1169) centre (-93.207, -232.0324) ccw
  circle A109 centre (-86.902, -84.1308) radius 5.588 projected
  circle A110 centre (-86.902, -84.1308) radius 12.6842
  circle A111 centre (-97.0281, -133.9113) radius 12.7176
  circle A112 centre (-63.595, -141.2799) radius 12.7
  spline S0 degree 4 poles (-85.584, -139.4585) (-82.6045, -141.2731) (-78.0776, -144.0197) (-76.3935, -137.6171) (-74.1957, -134.2859) knots 0 0 0 0 0 1 1 1 1 1
  line L42 (-33.8525, -134.6061) -> (-44.131, -133.8716)
  arc A113 (-44.131, -133.8716) -> (-54.8288, -148.877) centre (-44.9004, -144.6392) ccw
  line L43 (-54.8288, -148.877) -> (-51.872, -155.8042)
  arc A114 (-51.4648, -157.8766) -> (-51.872, -155.8042) centre (-56.5442, -157.7985) ccw
  arc A115 (-51.4648, -157.8766) -> (-45.5693, -167.6622) centre (-40.6711, -158.0425) ccw
  line L44 (-45.5693, -167.6622) -> (-40.3949, -170.2969)
  arc A116 (-40.3949, -170.2969) -> (-25.8769, -165.5754) centre (-35.4967, -160.6772) ccw
  line L45 (-25.8769, -165.5754) -> (-21.0127, -156.0224)
  arc A117 (-21.0127, -156.0224) -> (-23.3376, -143.167) centre (-30.6324, -151.1242) ccw
  arc A118 (-24.6142, -141.3269) -> (-23.3376, -143.167) centre (-19.9049, -139.4226) ccw
  arc A119 (-24.6142, -141.3269) -> (-33.8525, -134.6061) centre (-34.622, -145.3737) ccw
  circle A120 centre (-36.3661, -132.835) radius 1.5875
  point P0 (0, 0)
  point P1 (-79.4799, -141.0469)
  point P2 (-36.4792, -134.4184)
  point P3 (-35.3556, -131.6106)
  point P4 (-79.0435, -94.0873)
  point P5 (-88.3648, -96.7304)
  point P6 (-93.4457, -121.7087)
  point P7 (-74.1957, -134.2859)
  point P8 (-51.8713, -136.3967)
  dimension "d45" = 25.4
  dimension "d42" = 7.62
  dimension "d43" = 7.62
  dimension "d44" = 19.05
  dimension "d46" = 7.62
  dimension "d47" = 3.175
  constraints: 53 point on circle, 28 centre point, 26 end point, 3 coincident, 2 tangent, 46 other
  measures "d42" distance between parallel lines of L23 L33
  measures "d43" distance between parallel lines of L13 L36
  measures "d44" distance between parallel lines of L31 L39
  measures "d46" distance between parallel lines of L4 L42
  measures "d47" diameter of A120
extrude "Extrusion10" cut sketch "Sketch10" against normal blind 6.35 contours S0 A111 L39 A110 A96 L33 A120 L42 A113 A112 | A120
sketch "Sketch11" plane through (0, 0, 6.35) normal (0, 0, 1) x (1, 0, 0)
  line L0 (-44.131, -133.8716) -> (-53.8135, -133.1797)
  arc A0 (-51.8713, -136.3967) -> (-74.1957, -134.2859) centre (-63.595, -141.2799) ccw projected
  line L1 (-36.4792, -134.4184) -> (-44.131, -133.8716) projected
  arc A1 (-79.0435, -94.0873) -> (-76.0538, -98.0209) centre (-69.1823, -89.6953) ccw projected
  line L2 (-76.0538, -98.0209) -> (-35.3556, -131.6106) projected
  arc A2 (-36.4792, -134.4184) -> (-35.3556, -131.6106) centre (-36.3661, -132.835) ccw projected
  line L3 (-36.4792, -134.4184) -> (-44.131, -133.8716) projected
  arc A3 (-44.131, -133.8716) -> (-51.8713, -136.3967) centre (-44.9004, -144.6392) ccw projected
  arc A4 (-51.8713, -136.3967) -> (-74.1957, -134.2859) centre (-63.595, -141.2799) ccw projected
  arc A5 (-85.584, -139.4585) -> (-93.4457, -121.7087) centre (-97.0281, -133.9113) ccw projected
  line L4 (-93.4457, -121.7087) -> (-88.3648, -96.7304) projected
  arc A6 (-88.3648, -96.7304) -> (-79.0435, -94.0873) centre (-86.902, -84.1308) ccw projected
  arc A7 (-57.0315, -170.4891) -> (-48.9168, -167.9529) centre (-56.5442, -157.7985) ccw projected
  arc A8 (-45.5693, -167.6622) -> (-48.9168, -167.9529) centre (-47.0099, -170.4916) ccw projected
  line L5 (-45.5693, -167.6622) -> (-40.3949, -170.2969) projected
  arc A9 (-39.0062, -174.5669) -> (-40.3949, -170.2969) centre (-41.8356, -173.1263) ccw projected
  line L6 (-39.0062, -174.5669) -> (-46.1931, -188.6814) projected
  arc A10 (-49.6531, -190.3525) -> (-46.1931, -188.6814) centre (-49.0224, -187.2408) ccw projected
  arc A11 (-49.6531, -190.3525) -> (-53.7154, -190.1932) centre (-52.1756, -202.7997) ccw projected
  arc A12 (-56.7611, -188.774) -> (-53.7154, -190.1932) centre (-54.1004, -187.0416) ccw projected
  line L7 (-56.7611, -188.774) -> (-63.6057, -178.2615) projected
  line L8 (-44.8637, -152.8128) -> (-47.8206, -145.8856) projected
  arc A13 (-44.6741, -141.4723) -> (-47.8206, -145.8856) centre (-44.9004, -144.6392) ccw projected
  line L9 (-44.6741, -141.4723) -> (-34.3957, -142.2068) projected
  arc A14 (-31.6785, -144.1834) -> (-34.3957, -142.2068) centre (-34.622, -145.3737) ccw projected
  arc A15 (-31.6785, -144.1834) -> (-28.4869, -148.7838) centre (-19.9049, -139.4226) ccw projected
  arc A16 (-27.8031, -152.5648) -> (-28.4869, -148.7838) centre (-30.6324, -151.1242) ccw projected
  line L10 (-27.8031, -152.5648) -> (-32.6673, -162.1179) projected
  arc A17 (-36.9373, -163.5065) -> (-32.6673, -162.1179) centre (-35.4967, -160.6772) ccw projected
  line L11 (-36.9373, -163.5065) -> (-42.1117, -160.8718) projected
  arc A18 (-43.8457, -157.9937) -> (-42.1117, -160.8718) centre (-40.6711, -158.0425) ccw projected
  arc A19 (-43.8457, -157.9937) -> (-44.8637, -152.8128) centre (-56.5442, -157.7985) ccw projected
  arc A20 (-88.6501, -203.823) -> (-105.4512, -206.2136) centre (-93.207, -232.0324) ccw projected
  arc A21 (-109.9229, -202.7119) -> (-105.4512, -206.2136) centre (-106.8116, -203.3448) ccw projected
  line L12 (-109.9229, -202.7119) -> (-109.1463, -198.894) projected
  arc A22 (-106.2582, -196.3597) -> (-109.1463, -198.894) centre (-106.035, -199.5269) ccw projected
  arc A23 (-106.2582, -196.3597) -> (-98.2131, -192.7137) centre (-107.1508, -183.6911) ccw projected
  arc A24 (-94.9362, -191.9703) -> (-98.2131, -192.7137) centre (-95.9786, -194.9693) ccw projected
  line L13 (-94.9362, -191.9703) -> (-86.0453, -195.0607) projected
  arc A25 (-84.1415, -199.2432) -> (-86.0453, -195.0607) centre (-87.0877, -198.0597) ccw projected
  line L14 (-84.1415, -199.2432) -> (-85.1976, -201.8722) projected
  arc A26 (-88.6501, -203.823) -> (-85.1976, -201.8722) centre (-88.1438, -200.6887) ccw projected
  arc A27 (-28.8338, -52.5675) -> (-24.5423, -50.875) centre (-27.4885, -49.6916) ccw projected
  line L15 (-28.8338, -52.5675) -> (-62.2455, -36.9386) projected
  arc A28 (-64.0747, -34.1201) -> (-62.2455, -36.9386) centre (-60.9002, -34.0627) ccw projected
  arc A29 (-64.0747, -34.1201) -> (-69.5394, -23.9106) centre (-76.7726, -34.3495) ccw projected
  arc A30 (-70.5555, -19.8506) -> (-69.5394, -23.9106) centre (-67.7311, -21.3009) ccw projected
  arc A31 (-64.7921, -10.8233) -> (-70.5555, -19.8506) centre (-19.7161, -45.9556) ccw projected
  line L16 (-64.7921, -10.8233) -> (-52.5862, 4.8373) projected
  arc A32 (-46.9122, 2.7029) -> (-52.5862, 4.8373) centre (-50.0819, 2.8855) ccw projected
  arc A33 (-46.9122, 2.7029) -> (-23.4162, -40.7399) centre (0, 0) ccw projected
  arc A34 (-22.0522, -44.6761) -> (-23.4162, -40.7399) centre (-24.9984, -43.4926) ccw projected
  line L17 (-22.0522, -44.6761) -> (-24.5423, -50.875) projected
  arc A35 (-88.5384, -146.9458) -> (-92.3643, -145.7246) centre (-91.1992, -148.6781) ccw projected
  line L18 (-88.5384, -146.9458) -> (-60.6619, -189.7645) projected
  arc A36 (-61.0933, -193.7573) -> (-60.6619, -189.7645) centre (-63.3227, -191.4968) ccw projected
  arc A37 (-61.0933, -193.7573) -> (-61.1133, -193.7771) centre (-52.1756, -202.7997) ccw projected
  arc A38 (-64.3902, -194.5205) -> (-61.1133, -193.7771) centre (-63.3478, -191.5215) ccw projected
  line L19 (-64.3902, -194.5205) -> (-92.4345, -184.7727) projected
  arc A39 (-94.5438, -182.1572) -> (-92.4345, -184.7727) centre (-91.3921, -181.7737) ccw projected
  arc A40 (-94.5438, -182.1572) -> (-101.38, -172.378) centre (-107.1508, -183.6911) ccw projected
  arc A41 (-103.0485, -168.9169) -> (-101.38, -172.378) centre (-99.9372, -169.5497) ccw projected
  line L20 (-103.0485, -168.9169) -> (-99.0202, -149.1135) projected
  arc A42 (-96.1321, -146.5792) -> (-99.0202, -149.1135) centre (-95.909, -149.7463) ccw projected
  arc A43 (-96.1321, -146.5792) -> (-92.3643, -145.7246) centre (-97.0248, -133.9106) ccw projected
  arc A44 (-17.7611, -54.4364) -> (-16.1602, -58.4958) centre (-14.8149, -55.6198) ccw projected
  line L21 (-17.7611, -54.4364) -> (-14.9814, -47.5164) projected
  arc A45 (-11.2735, -45.6176) -> (-14.9814, -47.5164) centre (-12.0352, -48.6999) ccw projected
  arc A46 (-11.2735, -45.6176) -> (22.3352, -41.3425) centre (0, 0) ccw projected
  arc A47 (26.6737, -45.5765) -> (22.3352, -41.3425) centre (23.8443, -44.1359) ccw projected
  line L22 (26.6737, -45.5765) -> (18.3481, -61.9274) projected
  arc A48 (14.8881, -63.5984) -> (18.3481, -61.9274) centre (15.5187, -60.4867) ccw projected
  arc A49 (14.8881, -63.5984) -> (4.4031, -66.1517) centre (12.3657, -76.0454) ccw projected
  arc A50 (1.0672, -66.5541) -> (4.4031, -66.1517) centre (2.4124, -63.6782) ccw projected
  line L23 (1.0672, -66.5541) -> (-16.1602, -58.4958) projected
  arc A51 (-75.9854, -77.6347) -> (-81.1278, -72.8169) centre (-86.8987, -84.1301) ccw projected
  arc A52 (-82.7964, -69.3558) -> (-81.1278, -72.8169) centre (-79.6851, -69.9886) ccw projected
  line L24 (-82.7964, -69.3558) -> (-78.7681, -49.5524) projected
  arc A53 (-75.88, -47.0181) -> (-78.7681, -49.5524) centre (-75.6568, -50.1853) ccw projected
  arc A54 (-75.88, -47.0181) -> (-68.81, -44.2433) centre (-76.7726, -34.3495) ccw projected
  arc A55 (-65.4741, -43.8408) -> (-68.81, -44.2433) centre (-66.8194, -46.7167) ccw projected
  line L25 (-65.4741, -43.8408) -> (-13.0902, -68.3442) projected
  arc A56 (-14.1778, -74.3847) -> (-13.0902, -68.3442) centre (-14.4355, -71.2201) ccw projected
  line L26 (-14.1778, -74.3847) -> (-72.9993, -79.1754) projected
  arc A57 (-75.9854, -77.6347) -> (-72.9993, -79.1754) centre (-73.2571, -76.0109) ccw projected
  arc A58 (1.4524, -82.5408) -> (3.7836, -85.4069) centre (12.3657, -76.0454) ccw projected
  arc A59 (4.4674, -89.1879) -> (3.7836, -85.4069) centre (1.6381, -87.7473) ccw projected
  line L27 (4.4674, -89.1879) -> (-13.9226, -125.3045) projected
  arc A60 (-17.3825, -126.9756) -> (-13.9226, -125.3045) centre (-16.7519, -123.8638) ccw projected
  arc A61 (-17.3825, -126.9756) -> (-25.1437, -127.8534) centre (-19.9049, -139.4226) ccw projected
  arc A62 (-28.4744, -127.4098) -> (-25.1437, -127.8534) centre (-26.4534, -124.9611) ccw projected
  line L28 (-28.4744, -127.4098) -> (-71.2033, -92.144) projected
  arc A63 (-69.4401, -86.5307) -> (-71.2033, -92.144) centre (-69.1823, -89.6953) ccw projected
  line L29 (-69.4401, -86.5307) -> (-1.5337, -81.0001) projected
  arc A64 (1.4524, -82.5408) -> (-1.5337, -81.0001) centre (-1.2759, -84.1646) ccw projected
  arc A65 (-64.7826, -204.3336) -> (-60.7577, -212.1612) centre (-52.1756, -202.7997) ccw projected
  arc A66 (-60.0739, -215.9422) -> (-60.7577, -212.1612) centre (-62.9032, -214.5015) ccw projected
  line L30 (-60.0739, -215.9422) -> (-61.8764, -219.4822) projected
  arc A67 (-67.5559, -219.4407) -> (-61.8764, -219.4822) centre (-64.7057, -218.0416) ccw projected
  arc A68 (-67.5559, -219.4407) -> (-76.9832, -208.5096) centre (-93.207, -232.0324) ccw projected
  arc A69 (-78.1267, -204.7125) -> (-76.9832, -208.5096) centre (-75.1805, -205.896) ccw projected
  line L31 (-78.1267, -204.7125) -> (-76.8234, -201.468) projected
  arc A70 (-72.8348, -199.6524) -> (-76.8234, -201.468) centre (-73.8772, -202.6514) ccw projected
  line L32 (-72.8348, -199.6524) -> (-66.8919, -201.7181) projected
  arc A71 (-64.7826, -204.3336) -> (-66.8919, -201.7181) centre (-67.9343, -204.7171) ccw projected
  circle A72 centre (-19.9049, -139.4226) radius 5.588 projected
  circle A73 centre (-107.1541, -183.6919) radius 5.588 projected
  circle A74 centre (-86.902, -84.1308) radius 5.588 projected
  circle A75 centre (-56.5442, -157.7985) radius 6.731 projected
  line L33 (-98.5201, -236.7413) -> (-93.7862, -224.9565) projected
  arc A76 (-87.8938, -227.3235) -> (-93.7862, -224.9565) centre (-90.84, -226.14) ccw projected
  line L34 (-87.8938, -227.3235) -> (-92.6277, -239.1082) projected
  arc A77 (-98.5201, -236.7413) -> (-92.6277, -239.1082) centre (-95.5739, -237.9247) ccw projected
  circle A78 centre (0, 0) radius 13.4937 projected
  arc A79 (56.5867, -28.8131) -> (-50.0844, 39.0359) centre (0, 0) ccw projected
  line L35 (-50.0844, 39.0359) -> (-79.8174, 0.8875) projected
  arc A80 (-79.8174, 0.8875) -> (-94.3869, -30.7665) centre (-19.7161, -45.9556) ccw projected
  line L36 (-94.3869, -30.7665) -> (-133.6537, -223.8049) projected
  arc A81 (-133.6537, -223.8049) -> (-56.4256, -250.7609) centre (-93.207, -232.0324) ccw projected
  line L37 (-56.4256, -250.7609) -> (56.5867, -28.8131) projected
  circle A82 centre (-63.595, -141.2799) radius 6.731 projected
  arc A83 (-11.6087, -28.8683) -> (-9.2396, -22.9769) centre (-10.4059, -25.9299) ccw projected
  arc A84 (-9.2396, -22.9769) -> (-11.6087, -28.8683) centre (-10.4424, -25.9152) ccw projected
  arc A85 (26.36, 16.5315) -> (20.9805, 13.1578) centre (23.6598, 14.8613) ccw projected
  arc A86 (20.9805, 13.1578) -> (26.36, 16.5315) centre (23.6807, 14.828) ccw projected
  arc A87 (23.8681, -19.9613) -> (18.9971, -15.8876) centre (21.4452, -17.9094) ccw projected
  arc A88 (18.9971, -15.8876) -> (23.8681, -19.9613) centre (21.42, -17.9396) ccw projected
  arc A89 (-7.5767, 30.1783) -> (-6.0305, 24.0196) centre (-6.8227, 27.0942) ccw projected
  arc A90 (-6.0305, 24.0196) -> (-7.5767, 30.1783) centre (-6.7845, 27.1038) ccw projected
  arc A91 (-31.0426, 2.1197) -> (-24.7075, 1.6871) centre (-27.8764, 1.8838) ccw projected
  arc A92 (-24.7075, 1.6871) -> (-31.0426, 2.1197) centre (-27.8737, 1.9231) ccw projected
  circle A93 centre (-76.7759, -34.3502) radius 5.588 projected
  circle A94 centre (-97.0281, -133.9113) radius 5.588 projected
  circle A95 centre (12.3657, -76.0454) radius 5.588 projected
  circle A96 centre (-52.1756, -202.7997) radius 5.588 projected
  point P0 (0, 0)
  point P1 (-51.8713, -136.3967)
  point P2 (-44.131, -133.8716)
  constraints: 2 end point, 1 collinear, 1 point on circle, 2 other
extrude "Extrusion11" add sketch "Sketch11" against normal blind 6.35 contours A3 A0 L0